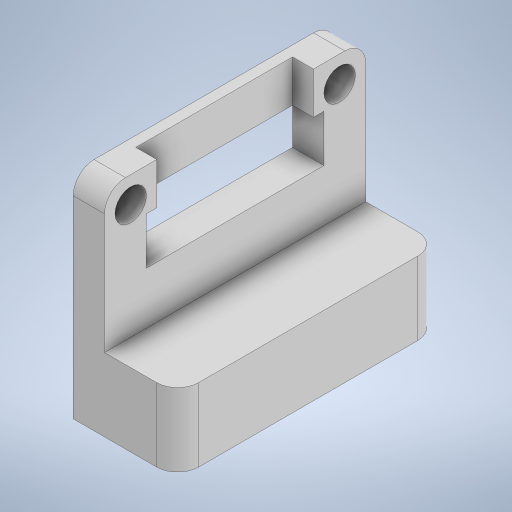
# Autodesk Inventor part: крепл_ЛД
Saved by Autodesk Inventor 2023 (Build 270158000, 158)
## iProperties
Created: 2025-12-19
Part Number: крепл_ЛД
Material: Типовые
Document SubType Name: Modeling
Designer: garin
Density: 1 g/cm^3
Appearance: По умолчанию
Author: garin
Autodesk Inventor part; units mm, degrees
ref_plane "YZ Plane" through (0, 0, 0) normal (1, 0, 0) x (0, 1, 0)
ref_plane "XZ Plane" through (0, 0, 0) normal (0, 1, 0) x (-1, 0, 0)
ref_plane "РабПлоскость7" through (-3, 0, 6) normal (-1, 0, 0) x (0, 0, 1)
sketch "Эскиз3" plane through (-3, 0, 6) normal (-1, 0, 0) x (0, 0, 1)
  line L0 (0, 0) -> (-12, 0) construction
  line L1 (0, 0) -> (0, 23.3031) construction
  line L2 (3, 0) -> (3, 3) construction
  circle A0 centre (-16, 19) radius 1.5
  circle A1 centre (4, 19) radius 1.5
  line L3 (-17.5, 19) -> (-18.5, 19)
  line L4 (-16, 20.5) -> (-16, 21.5)
  line L5 (-18.5, 21.5) -> (6.5, 21.5)
  line L6 (6.5, 21.5) -> (6.5, 13)
  line L7 (-18.5, 13) -> (-18.5, 21.5)
  line L8 (-18.5, 8) -> (-18.5, 13)
  line L9 (6.5, 8) -> (6.5, 13)
  line L10 (2.5, 17.5) -> (-14.5, 17.5)
  line L11 (-14.5, 17.5) -> (-14.5, 13)
  line L12 (-14.5, 13) -> (2.5, 13)
  line L13 (2.5, 13) -> (2.5, 17.5)
  line L14 (-3, 13) -> (-3, 8)
  line L15 (-9, 3) -> (-9, 13) projected
  line L16 (6.5, 8) -> (-4, 8)
  line L17 (-4, 8) -> (-4, 13)
  line L18 (-18.5, 8) -> (-8, 8)
  line L19 (-8, 8) -> (-8, 13)
  line L20 (-8, 8) -> (-4, 8)
  point P0 (-6, 0)
  point P1 (-9, 8)
  point P2 (-9, 8)
  dimension "d55" = 3
  dimension "d56" = 3
  dimension "d57" = 1
  dimension "d58" = 1
  dimension "d59" = 25
  dimension "d68" = 10.5
  dimension "d69" = 10.5
  constraints: 36 end point, 5 horizontal, 4 perpendicular, 3 parallel, 2 centre point, 2 point on circle, 2 vertical, 1 point on line
  measures "d55" diameter of A0
  measures "d56" diameter of A1
  measures "d57" distance of L3.start L3.end
  measures "d58" distance of L4.start L4.end
  measures "d59" distance of L6.end L7.start
  measures "d68" distance of L9.start L16.end
  measures "d69" distance of L8.start L18.end
extrude "Выдавливание10" add sketch "Эскиз3" against normal blind 3 contours A0 L4 L5 L6 L9 L16 L14 L12 L13 L10 L11 L15 L18 L8 L7 L3 | A0 L3 L7 L5 L4 | L15 L12 L19 L18 | L16 L17 L12 L14
extrude "Выдавливание12" add sketch "Эскиз3" against normal blind 3 contours L19 L12 L17 L20
sketch "Эскиз5" plane through (-3, 8, -12.5) normal (0, -1, 0) x (1, 0, 0)
  line L0 (7.899, 12.5) -> (3, 12.5) construction
  line L1 (0, 25) -> (10, 25)
  line L2 (10, 25) -> (10, 0)
  line L3 (10, 0) -> (0, 0)
  line L4 (0, 0) -> (0, 25)
  circle A0 centre (6.5, 4.4) radius 2.1
  line L5 (3, 25) -> (6.5, 25)
  line L6 (6.5, 25) -> (6.5, 0)
  circle A1 centre (6.5, 20.6) radius 2.1
  point P0 (8, 5.5)
  point P1 (6.5, 18.5)
  point P2 (6.5, 6.5)
  point P3 (6.5, 4.4)
  dimension "d94" = 10
  dimension "d95" = 25
  dimension "d96" = 4.2
  dimension "d102" = 3.5
  constraints: 14 end point, 5 point on line, 2 centre point, 2 horizontal, 2 parallel, 2 perpendicular, 1 coincident, 1 symmetric about line, 1 other
  measures "d94" distance of L2.end L3.end
  measures "d95" distance of L1.end L2.end
  measures "d96" diameter of A0
  measures "d102" distance of L5.start L5.end
extrude "Выдавливание13" [suppressed]
fillet "Сопряжение18" [suppressed]
fillet "Сопряжение19" radius 2 2 edges at (-1.5, 21.5, -12.5) (-1.5, 21.5, 12.5)
extrude "Выдавливание14" add sketch "Эскиз5" along normal blind 7
extrude "Выдавливание15" cut sketch "Эскиз5" against normal blind 6 from surface at 7 contours L6 A0 | A0 L6
fillet "Сопряжение20" radius 2 2 edges at (7, 4.5, -12.5) (7, 4.5, 12.5)
extrude "Выдавливание16" cut sketch "Эскиз5" against normal blind 6 from surface at 7 contours A1 L6 | L6 A1
sketch "Эскиз6" plane through (-3, 0, 6) normal (-1, 0, 0) x (0, 0, 1)
  point P0 (-6, 0)
sketch "Эскиз8" plane through (0, 0, 6) normal (1, 0, 0) x (0, 0, -1)
  circle A0 centre (-4, 19) radius 1.5 construction
  line L0 (-2.5, 19) -> (-1.5, 19) construction
  line L1 (-4.5, 21.5) -> (16.5, 21.5) projected
  line L2 (-2.5, 17.5) -> (14.5, 17.5) projected
  line L3 (-1.5, 21.5) -> (13.5, 21.5) construction
  line L4 (13.5, 21.5) -> (13.5, 17.5)
  line L5 (13.5, 17.5) -> (-1.5, 17.5) construction
  line L6 (-1.5, 17.5) -> (-1.5, 21.5)
  point P0 (6, 0)
  dimension "d105" = 1
  dimension "d106" = 15
  constraints: 10 end point, 2 horizontal, 2 parallel, 2 point on line, 1 horizontal alignment, 1 perpendicular, 1 other
  measures "d105" distance of L0.start L0.end
  measures "d106" distance of L4.end L5.end
extrude "Выдавливание17" cut sketch "Эскиз8" against normal blind 2
